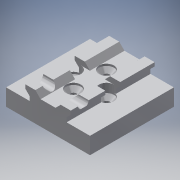
# Autodesk Inventor part: Gantry_Mount_Rail
Saved by Autodesk Inventor 2019 (Build 230136000, 136)
## iProperties
Created: 2021-01-31
Part Number: Gantry_Mount_Rail
Material: ABS Plastic
Document SubType Name: Modeling
Designer: zhanb
Density: 1.06 g/cm^3
Appearance: Smooth - White
Author: zhanb
Autodesk Inventor part; units mm, degrees
ref_plane "YZ Plane" through (0, 0, 0) normal (1, 0, 0) x (0, 1, 0)
ref_plane "XZ Plane" through (0, 0, 0) normal (0, 1, 0) x (-1, 0, 0)
ref_plane "XY Plane" through (0, 0, 0) normal (0, 0, 1) x (1, 0, 0)
sketch "Sketch1" plane through (0, 0, 0) normal (0, 1, 0) x (-1, 0, 0)
  line L0 (25.4, 25.4) -> (-25.4, 25.4)
  line L1 (-25.4, 25.4) -> (-25.4, -25.4)
  line L2 (-25.4, -25.4) -> (25.4, -25.4)
  line L3 (25.4, -25.4) -> (25.4, 25.4)
  line L4 (25.4, 25.4) -> (-25.4, -25.4) construction
  line L5 (-25.4, 25.4) -> (25.4, -25.4) construction
  point P0 (0, 0)
  dimension "d0" = 50.8
  dimension "d1" = 50.8
  constraints: 12 end point, 2 midpoint, 2 parallel, 1 horizontal, 1 perpendicular
  measures "d0" distance of L2.end L1.end
  measures "d1" distance of L1.end L0.end
extrude "Extrusion1" add sketch "Sketch1" along normal blind 10.16
sketch "Sketch2" plane through (-25.4, 0, 25.4) normal (0, 0, 1) x (1, 0, 0)
  line L0 (0, 10.16) -> (50.8, 10.16) projected
  line L1 (36.83, 10.16) -> (36.83, 12.7) construction
  line L2 (36.83, 12.7) -> (39.37, 15.24) construction
  line L3 (39.37, 15.24) -> (39.37, 17.78) construction
  line L4 (39.37, 17.78) -> (33.02, 17.78) construction
  line L5 (33.02, 17.78) -> (29.845, 14.605) construction
  line L6 (29.845, 14.605) -> (25.4, 14.605) construction
  line L7 (25.4, 14.605) -> (25.4, 10.16) construction
  line L8 (25.4, 10.16) -> (36.83, 10.16) construction
  line L9 (36.6316, 10.16) -> (36.6316, 12.7822)
  line L10 (36.6316, 12.7822) -> (39.1716, 15.3222)
  line L11 (39.1716, 15.3222) -> (39.1716, 17.5816)
  line L12 (39.1716, 17.5816) -> (33.1022, 17.5816)
  line L13 (33.1022, 17.5816) -> (29.9272, 14.4066)
  line L14 (29.9272, 14.4066) -> (25.4, 14.4066)
  line L15 (25.4, 10.16) -> (25.4, 14.4066)
  line L16 (25.4, 10.16) -> (36.6316, 10.16)
  point P0 (25.4, 0)
  dimension "d4" = 2.54
  dimension "d5" = 2.54
  dimension "d6" = 135
  dimension "d7" = 3.175
  dimension "d8" = 6.35
  dimension "d9" = 13.97
  dimension "d10" = 11.43
  dimension "d26" = 0.1984
  dimension "d27" = 0.1984
  dimension "d28" = 0.1984
  dimension "d29" = 0.1984
  dimension "d30" = 0.1984
  dimension "d31" = 0.1984
  constraints: 32 end point, 7 parallel, 3 perpendicular, 3 point on line, 2 collinear, 2 vertical, 1 midpoint
  measures "d4" distance of L1.start L1.end
  measures "d5" distance of L2.end L3.end
  measures "d6" angle of L6 L5
  measures "d7" horizontal distance of L4.end L5.end
  measures "d8" distance of L3.end L4.end
  measures "d9" distance between parallel lines of L7 L3
  measures "d10" distance between parallel lines of L7 L1
  measures "d26" distance between parallel lines of L6 L14
  measures "d27" distance between parallel lines of L5 L13
  measures "d28" distance between parallel lines of L4 L12
  measures "d29" distance between parallel lines of L11 L3
  measures "d30" distance between parallel lines of L10 L2
  measures "d31" distance between parallel lines of L9 L1
extrude "Extrusion2" add sketch "Sketch2" against normal up to surface (50.8 mm away)
mirror "Mirror1" about plane through (0, 10.16, 25.4) normal (-1, 0, 0) of "Extrusion2"
sketch "Sketch3" plane through (0, 0, 0) normal (0, -1, 0) x (1, 0, 0)
  line L0 (0, -10) -> (10, 0) construction
  line L1 (10, 0) -> (0, 10) construction
  line L2 (0, 10) -> (-10, 0) construction
  line L3 (-10, 0) -> (0, -10) construction
  line L4 (0, -10) -> (0, 10) construction
  line L5 (10, 0) -> (-10, 0) construction
  point P0 (0, 0)
  point P1 (-10, 0)
  dimension "d13" = 20
  constraints: 12 end point, 4 coincident, 2 midpoint, 2 parallel, 2 perpendicular, 1 horizontal
  measures "d13" distance of L0.start L1.end
hole "Hole1" at (0, 0, 10) at (-10, 0, 0) at (0, 0, -10) at (10, 0, 0) direction (0, 1, 0) diameter 4.2 end through all
sketch "Sketch4" plane through (4.3628, 14.4066, 25.4) normal (0, 1, 0) x (1, 0, 0)
  arc A0 (5.6372, 29.9) -> (5.6372, 20.9) centre (5.6372, 25.4) ccw
  circle A1 centre (-4.3628, 15.4) radius 4.5
  arc A2 (-14.3628, 29.9) -> (-14.3628, 20.9) centre (-14.3628, 25.4) ccw
  circle A3 centre (-4.3628, 35.4) radius 4.5
  line L0 (-14.3628, 20.9) -> (-18.1344, 20.9)
  line L1 (-18.1344, 20.9) -> (-18.1344, 29.9)
  line L2 (-18.1344, 29.9) -> (-14.3628, 29.9)
  line L3 (5.6372, 20.9) -> (9.4088, 20.9)
  line L4 (9.4088, 20.9) -> (9.4088, 29.9)
  line L5 (9.4088, 29.9) -> (5.6372, 29.9)
  arc A4 (5.6372, 20.9) -> (5.6372, 29.9) centre (5.6372, 25.4) ccw
  arc A5 (-14.3628, 20.9) -> (-14.3628, 29.9) centre (-14.3628, 25.4) ccw
  line L6 (9.4088, 0) -> (9.4088, 50.8) projected
  line L7 (-18.1344, 0) -> (-18.1344, 50.8) projected
  circle A6 centre (-4.3628, 15.4) radius 2.1 construction
  circle A7 centre (5.6372, 25.4) radius 2.1 construction
  circle A8 centre (-4.3628, 35.4) radius 2.1 construction
  circle A9 centre (-14.3628, 25.4) radius 2.1 construction
  line L8 (5.6372, 20.9) -> (-14.3628, 20.9)
  line L9 (-14.3628, 29.9) -> (5.6372, 29.9)
  dimension "d21" = 9
  constraints: 16 end point, 8 point on circle, 8 tangent, 6 centre point, 5 horizontal, 4 coincident, 4 concentric, 3 equal radius, 2 collinear, 2 perpendicular, 1 parallel
  measures "d21" diameter of A3
extrude "Extrusion3" cut sketch "Sketch4" along normal blind 10.16 contours A4 L4 A0 | L5 L4 A4 | A0 L8 A5 L9 | A4 L4 L3 | A5 A2 L1 | A2 L1 L2 | L0 L1 A2 | A1 | A3
extrude "Extrusion4" cut sketch "Sketch4" against normal blind 5.4 contours A4 L4 A0 | A4 L4 | A5 A2 L1 | L1 A2
extrude "Extrusion5" cut sketch "Sketch4" against normal up to surface (4.2466 mm away) contours A4 L4 A0 | L5 L4 A4 | A4 L4 L3 | A5 A2 L1 | A2 L1 L2 | L0 L1 A2
chamfer "Chamfer1" distance 2.4 angle 45 2 edges at (10, 9.0066, 2.1) (-10, 9.0066, 2.1)
extrude "Extrusion6" cut sketch "Sketch4" against normal blind 1.143 contours A1 | A3
chamfer "Chamfer2" distance 2.4 angle 45 2 edges at (0, 13.2636, 12.1) (0, 13.2636, -7.9)
sketch "Sketch5" plane through (-13.7716, 15.3222, 25.4) normal (-1, 0, 0) x (0, 0, 1)
  circle A0 centre (-7.62, 2.5446) radius 3.2639 construction
  line L0 (-10.8839, 2.5446) -> (-10.8839, 2.2594) construction
  line L1 (-10.8839, 2.2594) -> (-4.3686, 2.2594) construction
  line L2 (-10.8839, 2.2594) -> (-10.8839, 2.5446) construction
  line L3 (0, 2.2594) -> (-20.9, 2.2594) construction
  line L4 (0, 2.2594) -> (-20.9, 2.2594) construction
  line L5 (0, 2.2594) -> (-20.9, 2.2594) construction
  arc A1 (-10.8839, 2.5446) -> (-10.8714, 2.2594) centre (-7.62, 2.5446) ccw construction
  arc A2 (-4.3686, 2.2594) -> (-10.8839, 2.5446) centre (-7.62, 2.5446) ccw construction
  line L6 (-4.3686, 2.2594) -> (-10.8714, 2.2594) construction
  line L7 (-10.8714, 2.2594) -> (-10.8839, 2.2594) construction
  circle A3 centre (-7.62, 2.5467) radius 3.2639 projected
  point P0 (-25.4, -15.3222)
  dimension "d44" = 7.62
  dimension "d45" = 6.5278
  constraints: 10 end point, 6 point on circle, 3 centre point, 3 horizontal, 3 point on line, 2 tangent, 1 coincident, 1 collinear, 1 vertical
  measures "d44" horizontal distance of L3.start A0.centre
  measures "d45" diameter of A0
extrude "Extrusion7" cut sketch "Sketch5" against normal through all
equation "\"d27\" = d26"
equation "\"d28\" = d26"
equation "\"d29\" = d26"
equation "\"d30\" = d26"
equation "\"d31\" = d26"
body "Solid1"
